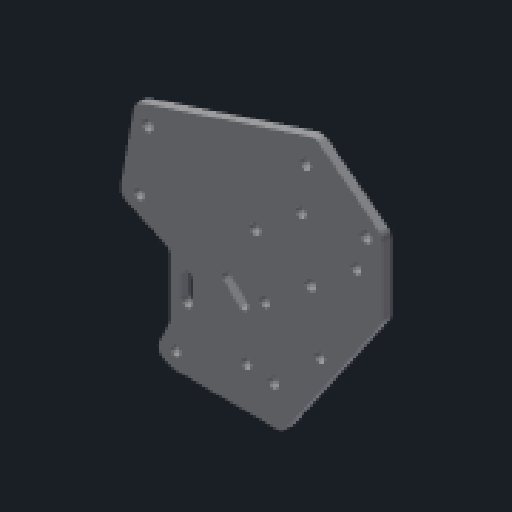
# Autodesk Inventor part: LegInsideConnector
Saved by Autodesk Inventor 2025.2 (Build 292293000, 293)
## iProperties
Created: 2025-10-14
Part Number: LegInsideConnector
Material: Generic
Document SubType Name: Sheet Metal
Designer: valer
Density: 1 g/cm^3
Sheet Metal Rule: Default
Appearance: Default
Author: valer
Autodesk Inventor part; units mm, degrees
ref_plane "YZ Plane" through (0, 0, 0) normal (1, 0, 0) x (0, 1, 0)
ref_plane "XZ Plane" through (0, 0, 0) normal (0, 1, 0) x (-1, 0, 0)
ref_plane "XY Plane" through (0, 0, 0) normal (0, 0, 1) x (1, 0, 0)
sketch "Base" plane through (0, 0, 0) normal (0, 0, 1) x (1, 0, 0)
  circle A0 centre (-32.6724, 68.8202) radius 3
  circle A1 centre (8.9104, 82.9577) radius 3
  circle A2 centre (24.8709, 81.2906) radius 3
  arc A3 (-29.0654, 97.1108) -> (-22.7155, 97.0843) centre (-25.8905, 97.0976) ccw
  line L0 (-22.6625, 109.7842) -> (-22.7155, 97.0843)
  arc A4 (-22.6625, 109.7842) -> (-29.0124, 109.8107) centre (-25.8375, 109.7974) ccw
  line L1 (-29.0654, 97.1108) -> (-29.0124, 109.8107)
  arc A5 (-0.0115, 123.2106) -> (-4.3609, 118.584) centre (-2.1862, 120.8973) ccw
  line L2 (4.8922, 109.8852) -> (-4.3609, 118.584)
  line L3 (-0.0115, 123.2106) -> (9.2416, 114.5118)
  arc A6 (4.8922, 109.8852) -> (9.2416, 114.5118) centre (7.0669, 112.1985) ccw
  circle A7 centre (-54.1178, 137.76) radius 3.175
  circle A8 centre (-49.1635, 174.9595) radius 3.175
  circle A9 centre (78.9408, 182.4168) radius 3.175
  circle A10 centre (43.6326, 201.5827) radius 3.175
  circle A11 centre (51.9282, 107.4544) radius 3.175
  circle A12 centre (19.6295, 119.7375) radius 3.175
  circle A13 centre (14.1176, 153.8506) radius 3.175
  circle A14 centre (46.4163, 141.5674) radius 3.175
  circle A15 centre (78.715, 129.2843) radius 3.175 construction
  circle A16 centre (73.2032, 163.3974) radius 3.175
  circle A17 centre (40.9045, 175.6805) radius 3.175
  line L4 (-65.2677, 131.7848) -> (-56.6187, 183.0321)
  line L5 (-56.6187, 183.0321) -> (49.256, 217.9127)
  line L6 (49.256, 217.9127) -> (88.9408, 187.3359)
  line L7 (88.9408, 187.3359) -> (88.9408, 143.386)
  line L8 (88.9408, 143.386) -> (30.2658, 58.5574)
  line L9 (30.2658, 58.5574) -> (-34.8221, 58.8291)
  line L10 (-34.8221, 58.8291) -> (-44.2886, 63.0531)
  line L11 (-44.2886, 63.0531) -> (-35.9547, 81.7302)
  line L12 (-35.9547, 81.7302) -> (-35.8006, 118.6364)
  line L13 (-35.8006, 118.6364) -> (-65.2677, 131.7848)
  line L14 (-80.6316, -18.3957) -> (-39.2676, 74.3056) construction
  line L15 (106.2259, 158.4266) -> (73.8476, 111.6161) construction
  line L16 (52.3387, 226.8078) -> (103.9962, 187.0062) construction
  line L17 (106.4643, 182.257) -> (107.3472, 162.3198) construction
  line L18 (-70.1334, 189.3917) -> (46.4761, 227.8089) construction
  line L19 (-90.3471, 89.9733) -> (-74.4079, 184.4173) construction
  point P0 (0, 0)
  dimension "d0" = 10
  dimension "d1" = 10
  dimension "d2" = 10
  dimension "d3" = 10
  dimension "d4" = 10
  dimension "d6" = 10
  dimension "d7" = 10
  dimension "d8" = 10
  dimension "d9" = 10
  measures "d0" distance from line of L9 A0.centre
  measures "d1" distance from line of L8 A11.centre
  measures "d2" distance from line of L12 A3.centre
  measures "d3" distance from line of A7.centre L4
  measures "d4" distance from line of L5 A8.centre
  measures "d6" distance from line of L6 A9.centre
  measures "d7" distance from line of A0.centre L10
  measures "d8" distance from line of L13 A7.centre
  measures "d9" distance from line of L7 A9.centre
extrude "Plate1" add sketch "Base" along normal blind 5
fillet "FilletsFeature" radius 6 10 edges at (-56.6187, 183.0321, 2.5) (49.256, 217.9127, 2.5) (88.9408, 187.3359, 2.5) (88.9408, 143.386, 2.5) (30.2658, 58.5574, 2.5) (-34.8221, 58.8291, 2.5) (-44.2886, 63.0531, 2.5) (-35.9547, 81.7302, 2.5) (-35.8006, 118.6364, 2.5) (-65.2677, 131.7848, 2.5)
equation "\"d1\" = d0"
equation "\"d2\" = d0"
equation "\"d3\" = d0"
equation "\"d4\" = d0"
equation "\"d6\" = d0"
equation "\"d7\" = d0"
equation "\"d8\" = d0"
equation "\"d9\" = d0"
equation "\"d10\" = Thickness"
equation "\"BendRadius\" = Thickness"
equation "\"BendReliefWidth\" = Thickness"
equation "\"BendReliefDepth\" = 0.5 * Thickness"
equation "\"TransitionRadius\" = BendRadius"
equation "\"JacobiRadiusSize\" = BendRadius"
equation "\"GapSize\" = Thickness"
equation "\"Thickness\" = 5"
body "Solid1"
